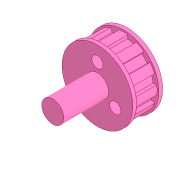
# Autodesk Inventor part: Nut3
Saved by Autodesk Inventor 2022.5 (Build 265521000, 521)
## iProperties
Created: 2011-08-19
Part Number: Nut3
Document SubType Name: Modeling
Designer: nguyenducthang
Density: 1 g/cm^3
Mass: 2.08832 g
Surface Area: 19.6745 cm^2
Volume: 2.08832 cm^3
Material: Generic
Appearance: Pink
Author: nguyenducthang
Autodesk Inventor part; units mm, degrees
ref_plane "YZ Plane" through (0, 0, 0) normal (1, 0, 0) x (0, 1, 0)
ref_plane "XZ Plane" through (0, 0, 0) normal (0, 1, 0) x (-1, 0, 0)
ref_plane "XY Plane" through (0, 0, 0) normal (0, 0, 1) x (1, 0, 0)
sketch "Sketch19" plane through (0, 0, 0) normal (1, 0, 0) x (0, 1, 0)
  line L0 (0, 0) -> (3, 0)
  line L1 (3, 0) -> (3, -4)
  line L2 (3, -4) -> (9.5, -4)
  line L3 (9.5, -4) -> (9.5, 0) construction
  line L4 (9.5, 0) -> (3, 0) construction
  line L5 (9.5, -3) -> (8, -3)
  line L6 (8, -3) -> (8, 0)
  line L7 (0, 0) -> (0, -7.3886)
  line L8 (3, 0) -> (3, 4)
  line L9 (3, 4) -> (9.5, 4)
  line L10 (9.5, 4) -> (9.5, 0) construction
  line L11 (9.5, 3) -> (8, 3)
  line L12 (8, 3) -> (8, 0)
  line L13 (9.5, 4) -> (9.5, 3)
  line L14 (9.5, -3) -> (9.5, -4)
  dimension "d111" = 1
  dimension "d113" = 3
  dimension "d119" = 6
  dimension "d120" = 1.5
  dimension "d121" = 8
  constraints: 30 end point, 6 perpendicular, 4 point on line, 4 symmetric about line, 2 collinear, 1 horizontal, 1 vertical
  measures "d111" distance from line of L2 L5.start
  measures "d113" distance between parallel lines of L7 L1
  measures "d119" distance between parallel lines of L5 L11
  measures "d120" distance between parallel lines of L12 L10
  measures "d121" distance between parallel lines of L7 L6
revolve "Revolution4" add sketch "Sketch19" angle 360 about axis through (0, 0, 0) along (0, 0, -1)
sketch "Sketch20" plane through (0, 0, -4) normal (0, 0, -1) x (-1, 0, 0)
  circle A0 centre (0, 0) radius 3 projected
  circle A1 centre (0, 0) radius 2.96
  dimension "d116" = 0.04
  constraints: 1 centre point
  measures "d116" radial gap between concentric circles of A0 A1
extrude "Extrusion16" add sketch "Sketch20" against normal blind 20 contours A1
sketch "Sketch21" plane through (0, 0, 4) normal (0, 0, 1) x (1, 0, 0)
  circle A0 centre (0, 0) radius 8 projected
  circle A1 centre (0, 0) radius 2.96 projected
  circle A2 centre (0, 0) radius 2.96 construction
  line L0 (0, 0) -> (0, 3) construction
  circle A3 centre (0, 0) radius 3 construction
  line L1 (0, 3) -> (0, 8) construction
  circle A4 centre (0, 5.5) radius 1.5
  dimension "d122" = 3
  constraints: 4 end point, 2 vertical alignment, 1 centre point, 1 midpoint, 1 point on line, 1 vertical, 2 other
  measures "d122" diameter of A4
extrude "Extrusion17" cut sketch "Sketch21" against normal through all contours A4
pattern_circular "Circular Pattern1" count 3 over 360 about axis through (0, 0, -4) along (0, 0, 1) of "Extrusion17"
sketch "Sketch22" plane through (0, 0, -3) normal (0, 0, 1) x (1, 0, 0)
  circle A0 centre (0, 0) radius 8 projected
  circle A1 centre (0, 0) radius 9
  line L0 (0, 0) -> (-1.1747, 8.923) construction
  line L1 (-1.1747, 8.923) -> (1.1747, 8.923) construction
  circle A2 centre (0, 0) radius 8 construction
  line L2 (1.1747, 8.923) -> (0, 0) construction
  line L3 (-1.0442, 7.9316) -> (-1.1747, 8.923)
  line L4 (1.0442, 7.9316) -> (1.1747, 8.923)
  dimension "d128" = 1
  dimension "d129" = 15
  constraints: 10 end point, 4 point on circle, 2 collinear, 2 point on line, 1 centre point, 1 coincident, 1 horizontal
  measures "d128" radial gap between concentric circles of A0 A1
  measures "d129" angle of L2 L0
extrude "Extrusion18" add sketch "Sketch22" along normal up to surface (6 mm away) contours A0 L3 A1 L4 picked at (0.1163, 8.6584)
pattern_circular "Circular Pattern2" count 12 over 360 about axis through (0, 0, -4) along (0, 0, 1) of "Extrusion18"
body "Solid2"
